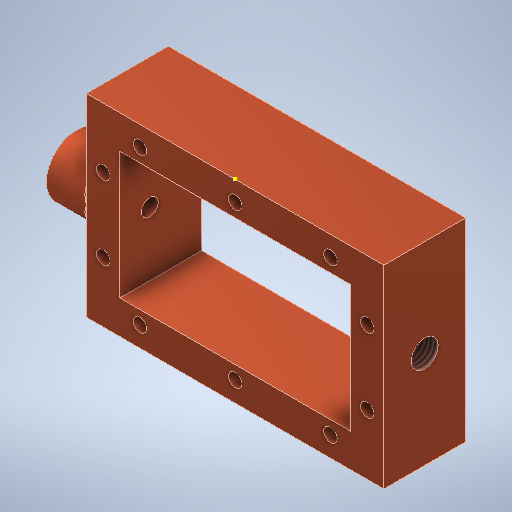
# Autodesk Inventor part: 1152_body
Saved by Autodesk Inventor 2025.1 (Build 291241000, 241)
## iProperties
Created: 2024-06-07
Part Number: 1152_body
Material: Kupfer
Document SubType Name: Modeling
Designer: ffogue
Density: 8.94 g/cm^3
Appearance: Kupfer - satiniert
Author: ffogue
Autodesk Inventor part; units mm, degrees
ref_plane "XZ Plane" through (0, 0, 0) normal (0, 1, 0) x (-1, 0, 0)
sketch "Skizze1" plane through (0, 0, 0) normal (0, 1, 0) x (-1, 0, 0)
  line L0 (44.5, -29) -> (-44.5, -29)
  line L1 (-44.5, -29) -> (-44.5, 29)
  line L2 (-44.5, 29) -> (44.5, 29)
  line L3 (44.5, 29) -> (44.5, -29)
  line L4 (44.5, -29) -> (-44.5, 29) construction
  line L5 (-44.5, -29) -> (44.5, 29) construction
  line L6 (29.2256, -19.0459) -> (-29.2256, 19.0459) construction
  line L7 (-26.1368, -16.746) -> (26.1368, 16.746) construction
  point P0 (0, 0)
  dimension "d0" = 89
  dimension "d1" = 58
  constraints: 16 end point, 4 midpoint, 2 parallel, 1 horizontal, 1 perpendicular, 1 point on line
  measures "d0" distance of L1.end L2.end
  measures "d1" distance between parallel lines of L0 L2
extrude "Extrusion1" add sketch "Skizze1" along normal blind 24.5
sketch "Skizze2" plane through (0, 24.5, 0) normal (0, 1, 0) x (1, 0, 0)
  line L0 (34.5, 19) -> (-34.5, 19)
  line L1 (-34.5, 19) -> (-34.5, -19)
  line L2 (-34.5, -19) -> (34.5, -19)
  line L3 (34.5, -19) -> (34.5, 19)
  line L4 (34.5, 19) -> (-34.5, -19) construction
  line L5 (-34.5, 19) -> (34.5, -19) construction
  line L6 (44.5, -29) -> (44.5, 29) projected
  point P0 (0, 0)
  dimension "d4" = 38
  dimension "d5" = 10
  constraints: 12 end point, 2 midpoint, 2 parallel, 1 horizontal, 1 perpendicular
  measures "d4" distance between parallel lines of L2 L0
  measures "d5" distance between parallel lines of L6 L3
extrude "Extrusion2" cut sketch "Skizze2" against normal up to surface (24.5 mm away)
sketch "Skizze3" plane through (-44.5, 0, -29) normal (-1, 0, 0) x (0, 0, 1)
  circle A0 centre (29, 9) radius 9
  line L0 (0, 0) -> (0, 24.5) projected
  line L1 (0, 0) -> (58, 0) projected
  point P0 (29, 0)
  point P1 (0, 12.25)
  point P2 (29, 0)
  dimension "d8" = 18
  dimension "d19" = 9
  constraints: 2 midpoint, 1 centre point, 1 vertical alignment
  measures "d8" diameter of A0
  measures "d19" distance from line of L1 A0.centre
extrude "Extrusion3" add sketch "Skizze3" along normal blind 12
sketch "Skizze4" plane through (-56.5, 9, 0) normal (-1, 0, 0) x (0, 0, 1)
  circle A0 centre (0, 0) radius 9 projected
  point P0 (0, -9)
  constraints: 1 coincident
hole "Bohrung1" at (-56.5, 9, 0) direction (1, 0, 0) diameter 5 depth 22 counterbore diameter 10 counterbore depth 17
fillet "Rundung1" radius 1 2 edges at (-44.5, 15.364, -6.364) (-44.5, 2.636, 6.364)
sketch "Skizze5" plane through (-44.5, 0, 29) normal (0, 0, 1) x (1, 0, 0)
  point P0 (44.5, 0)
sketch "Skizze6" plane through (44.5, 0, 29) normal (1, 0, 0) x (0, 0, -1)
  circle A0 centre (29, 12.25) radius 4
  line L0 (58, 0) -> (58, 24.5) projected
  line L1 (0, 0) -> (58, 0) projected
  point P0 (29, 0)
  point P1 (58, 12.25)
  point P2 (29, 0)
  dimension "d20" = 8
  constraints: 2 midpoint, 1 centre point, 1 horizontal alignment, 1 vertical alignment
  measures "d20" diameter of A0
extrude "Extrusion4" cut sketch "Skizze6" against normal up to surface (10 mm away)
ref_plane "Arbeitsebene1" through (0, 0, 0) normal (0, 0, 1) x (1, 0, 0)
thread "Gewinde3" size "M8x1.25" class "6H" standard "ISO Metric profile" length 18
sketch "Skizze9" plane through (0, 0, 0) normal (0, -1, 0) x (1, 0, 0)
  line L0 (-44.5, -29) -> (-44.5, -4.3589) projected
  line L1 (44.5, -29) -> (-44.5, -29) projected
  line L2 (44.5, 29) -> (44.5, -29) projected
  point P0 (0, 0)
  point P1 (-44.5, -16.6794)
  point P2 (-28.5, -23)
  point P3 (28.5, -23)
  point P4 (0, -23)
  dimension "d63" = 16
  dimension "d64" = 16
  constraints: 2 horizontal alignment, 1 midpoint, 1 vertical alignment
  measures "d63" distance from line of L0 point (-28.5, -23)
  measures "d64" distance from line of L2 point (28.5, -23)
hole "Bohrung2" at (-28.5, 0, -23) at (28.5, 0, -23) at (0, 0, -23) direction (0, 1, 0) diameter 4 end through all
mirror "Spiegeln3" about plane through (0, 0, 0) normal (0, 0, 1) of "Bohrung2"
sketch "Skizze10" plane through (0, 0, 0) normal (0, -1, 0) x (1, 0, 0)
  line L0 (44.5, 29) -> (44.5, -29) projected
  point P0 (0, 0)
  point P1 (39.5, 11)
  point P2 (39.5, -11)
  point P3 (44.5, 0)
  point P4 (44.5, 0)
  dimension "d60" = 5
  dimension "d72" = 11
  dimension "d73" = 11
  constraints: 2 midpoint, 1 vertical alignment
  measures "d60" distance from line of L0 point (39.5, 11)
  measures "d72" vertical distance of point (44.5, 0) point (39.5, -11)
  measures "d73" vertical distance of point (44.5, 0) point (39.5, 11)
ref_plane "Arbeitsebene3" through (0, 0, 0) normal (1, 0, 0) x (0, 1, 0)
hole "Hole4" at (39.5, 0, -11) at (39.5, 0, 11) direction (0, 1, 0) diameter 4 depth 24.5
mirror "Mirror5" about plane through (0, 0, 0) normal (1, 0, 0) of "Hole4"
equation "\"d64\" = d63"
